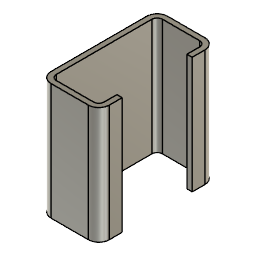
RC-100×50×20×4.5 (Autodesk Fusion 360 design; units mm, degrees)
Autodesk Fusion 360 part; units mm, degrees
sketch "スケッチ1" plane through (0, 0, 0) normal (0, 0, 1) x (1, 0, 0)
  line L0 (213.0702, 173.7996) -> (213.0702, 91.7996)
  line L1 (208.5702, 173.7996) -> (208.5702, 91.7996)
  arc A0 (249.5702, 82.7996) -> (258.5702, 91.7996) centre (249.5702, 91.7996) ccw
  arc A1 (249.5702, 87.2996) -> (254.0702, 91.7996) centre (249.5702, 91.7996) ccw
  line L2 (249.5702, 82.7996) -> (217.5702, 82.7996)
  line L3 (217.5702, 87.2996) -> (249.5702, 87.2996)
  arc A2 (208.5702, 91.7996) -> (217.5702, 82.7996) centre (217.5702, 91.7996) ccw
  arc A3 (213.0702, 91.7996) -> (217.5702, 87.2996) centre (217.5702, 91.7996) ccw
  line L4 (254.0702, 91.7996) -> (254.0702, 102.7996)
  line L5 (258.5702, 91.7996) -> (258.5702, 102.7996)
  line L6 (258.5702, 102.7996) -> (254.0702, 102.7996)
  arc A4 (258.5702, 173.7996) -> (249.5702, 182.7996) centre (249.5702, 173.7996) ccw
  arc A5 (254.0702, 173.7996) -> (249.5702, 178.2996) centre (249.5702, 173.7996) ccw
  arc A6 (217.5702, 182.7996) -> (208.5702, 173.7996) centre (217.5702, 173.7996) ccw
  arc A7 (217.5702, 178.2996) -> (213.0702, 173.7996) centre (217.5702, 173.7996) ccw
  line L7 (217.5702, 178.2996) -> (249.5702, 178.2996)
  line L8 (217.5702, 182.7996) -> (249.5702, 182.7996)
  line L9 (258.5702, 173.7996) -> (258.5702, 162.7996)
  line L10 (254.0702, 173.7996) -> (254.0702, 162.7996)
  line L11 (254.0702, 162.7996) -> (258.5702, 162.7996)
  point P0 (208.5702, 182.7996)
extrude "押し出し1" add sketch "スケッチ1" along normal blind 100
